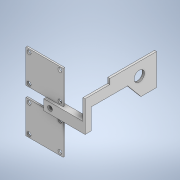
# Autodesk Inventor part: Shelf_half
Saved by Autodesk Inventor 2020.2 (Build 242310000, 310)
## iProperties
Created: 2020-02-18
Part Number: Shelf_half
Material: Generic
Document SubType Name: Modeling
Designer: ColinP
Density: 1 g/cm^3
Appearance: Default
Author: ColinP
Autodesk Inventor part; units mm, degrees
ref_plane "YZ Plane" through (0, 0, 0) normal (1, 0, 0) x (0, 1, 0)
ref_plane "XZ Plane" through (0, 0, 0) normal (0, 1, 0) x (-1, 0, 0)
ref_plane "XY Plane" through (0, 0, 0) normal (0, 0, 1) x (1, 0, 0)
sketch "Sketch14" plane through (0, 0, 0) normal (0, 0, 1) x (1, 0, 0)
  line L0 (0, 0) -> (-6.08, 0)
  line L1 (-6.08, 0) -> (0, 0)
  line L2 (0, 0) -> (6.08, 0)
  line L3 (-6.08, 0) -> (-6.08, 5)
  line L4 (-6.08, 0) -> (-1.08, 0) construction
  line L5 (-6.08, 5) -> (6.08, 5)
  line L6 (6.08, 5) -> (6.08, -5)
  line L7 (6.08, -5) -> (-6.08, -5)
  line L8 (-6.08, -5) -> (-6.08, 5)
  dimension "d66" = 6.08
  dimension "d67" = 6.08
  dimension "d68" = 5
  dimension "d69" = 90
  dimension "d70" = 12.16
  dimension "d71" = 10
  constraints: 18 end point, 3 equal length, 3 horizontal, 2 perpendicular, 1 point on line, 1 vertical
  measures "d66" distance of L0.start L0.end
  measures "d67" distance of L0.start L2.end
  measures "d68" distance of L0.end L3.end
  measures "d69" angle of L4 L3
  measures "d70" distance of L6.end L7.end
  measures "d71" distance of L5.end L6.end
extrude "Extrusion7" add sketch "Sketch14" along normal blind 2
sketch "Sketch15" plane through (0, 0, 2) normal (0, 0, 1) x (1, 0, 0)
  circle A0 centre (0, 0) radius 1.0665
  constraints: 1 centre point, 1 coincident
hole "Hole4" at (0, 0, 2) direction (0, 0, -1) diameter 4.5 end through all clearance for "Flat Head Machine Screw" size "M4" standard "Ansi Metric M Profile"
sketch "Sketch16" plane through (0, 0, 2) normal (0, 0, 1) x (1, 0, 0)
  line L0 (6.08, 5) -> (-6.08, 5) projected
  line L1 (0, 5) -> (10, 5)
  line L2 (10, 5) -> (-25.7, 5)
  line L3 (-25.7, 5) -> (-25.7, 37.05)
  line L4 (-25.7, 37.05) -> (10, 37.05)
  line L5 (10, 37.05) -> (10, 5)
  line L6 (-6.08, -5) -> (6.08, -5) projected
  line L7 (0, -5) -> (10, -5)
  line L8 (10, -5) -> (-25.7, -5)
  line L9 (-25.7, -5) -> (-25.7, -37.05)
  line L10 (-25.7, -37.05) -> (10, -37.05)
  line L11 (10, -37.05) -> (10, -5)
  line L12 (-25.7, 37.05) -> (-22.7, 37.05)
  line L13 (-22.7, 37.05) -> (-22.7, 34.05)
  line L14 (-22.7, 34.05) -> (-25.7, 34.05)
  line L15 (-25.7, 34.05) -> (-25.7, 37.05)
  line L16 (-22.7, 34.05) -> (7, 34.05)
  line L17 (7, 34.05) -> (7, 8)
  line L18 (7, 8) -> (-22.7, 8)
  line L19 (-22.7, 8) -> (-22.7, 34.05)
  line L20 (-25.7, -37.05) -> (-22.7, -37.05)
  line L21 (-22.7, -37.05) -> (-22.7, -34.05)
  line L22 (-22.7, -34.05) -> (-25.7, -34.05)
  line L23 (-25.7, -34.05) -> (-25.7, -37.05)
  line L24 (-22.7, -34.05) -> (7, -34.05)
  line L25 (7, -34.05) -> (7, -8)
  line L26 (7, -8) -> (-22.7, -8)
  line L27 (-22.7, -8) -> (-22.7, -34.05)
  line L28 (-25.7, -5) -> (10, -5)
  line L29 (10, -5) -> (10, -37.05)
  line L30 (10, -37.05) -> (-25.7, -37.05)
  line L31 (-25.7, -37.05) -> (-25.7, -5)
  point P0 (0, 0)
  dimension "d81" = 10
  dimension "d82" = 35.7
  dimension "d83" = 32.05
  dimension "d84" = 35.7
  dimension "d85" = 32.05
  dimension "d86" = 3
  dimension "d87" = 3
  dimension "d88" = 29.7
  dimension "d89" = 26.05
  dimension "d90" = 3
  dimension "d91" = 3
  dimension "d92" = 29.7
  dimension "d93" = 26.05
  dimension "d172" = 10
  constraints: 60 end point, 14 parallel, 9 horizontal, 7 perpendicular, 2 midpoint
  measures "d81" distance of L1.start L1.end
  measures "d82" distance of L3.end L4.end
  measures "d83" distance of L2.end L3.end
  measures "d84" distance of L10.end L9.end
  measures "d85" distance of L9.end L8.end
  measures "d86" distance of L13.end L14.end
  measures "d87" distance of L12.end L13.end
  measures "d88" distance of L17.end L18.end
  measures "d89" distance of L16.end L17.end
  measures "d90" distance of L22.end L21.end
  measures "d91" distance of L21.end L20.end
  measures "d92" distance of L26.end L25.end
  measures "d93" distance of L25.end L24.end
  measures "d172" distance from line of L7.start L11
extrude "Extrusion8" add sketch "Sketch16" along normal blind 1.5 contours L16 L17 L18 L19 | L0 L2 L3 L14 L13 L4 L5 L1 | L13 L14 L3 L4 | L27 L26 L25 L24 | L6 L7 L11 L10 L21 L22 L9 L8 | L22 L21 L10 L9
hole "Hole5" at (-22.7, 34.05, 2) at (-22.7, 8, 2) at (7, 8, 2) at (7, 34.05, 2) at (7, -8, 2) at (7, -34.05, 2) at (-22.7, -34.05, 2) at (-22.7, -8, 2) direction (0, 0, 1) diameter 3.9 end through all clearance for "Flat Head Machine Screw" size "M3.5" standard "Ansi Metric M Profile"
sketch "Sketch17" plane through (0, 0, 2) normal (0, 0, 1) x (1, 0, 0)
  circle A0 centre (0, 0) radius 2.25 projected
  line L0 (6.08, -5) -> (6.08, 5) projected
  line L1 (6.08, 5) -> (-6.08, 5) projected
  line L2 (-6.08, 5) -> (-6.08, -5) projected
  line L3 (-6.08, -5) -> (6.08, -5) projected
extrude "Extrusion9" add sketch "Sketch17" along normal blind 4
sketch "Sketch18" plane through (6.08, -5, 0) normal (1, 0, 0) x (0, 0, -1)
  line L0 (0, 0) -> (0, 10) projected
  line L1 (0, 10) -> (-2, 10) projected
  line L2 (-3.5, 10) -> (-2, 10) projected
  line L3 (-3.5, 10) -> (-6, 10) projected
  line L4 (-6, 0) -> (-6, 10) projected
  line L5 (-3.5, 0) -> (-6, 0) projected
  line L6 (-2, 0) -> (-3.5, 0) projected
  line L7 (0, 0) -> (-2, 0) projected
  point P0 (0, 5)
extrude "Extrusion10" add sketch "Sketch18" along normal blind 35
sketch "Sketch19" plane through (41.08, -5, 0) normal (1, 0, 0) x (0, 0, -1)
  line L0 (-6, 10) -> (-6, 0) projected
  line L1 (-6, 0) -> (-16, 0)
  line L2 (-16, 0) -> (-16, 50)
  line L3 (-16, 50) -> (29, 50)
  line L4 (29, 50) -> (29, 25)
  line L5 (29, 25) -> (0, 10)
  line L6 (0, 10) -> (0, 0) projected
  line L7 (0, 10) -> (0, 0)
  line L8 (0, 0) -> (-6, 0)
  point P0 (0, 5)
  dimension "d107" = 10
  dimension "d108" = 50
  dimension "d109" = 90
  dimension "d110" = 45
  dimension "d111" = 90
  dimension "d112" = 25
  constraints: 14 end point, 3 perpendicular, 1 horizontal, 1 parallel, 1 vertical
  measures "d107" distance of L0.end L1.end
  measures "d108" distance of L1.end L2.end
  measures "d109" angle of L1 L2
  measures "d110" distance of L2.end L3.end
  measures "d111" angle of L2 L3
  measures "d112" distance of L3.end L4.end
extrude "Extrusion11" add sketch "Sketch19" along normal blind 2.5
sketch "Sketch21" plane through (43.58, -5, 0) normal (1, 0, 0) x (0, 0, -1)
  line L0 (-3.5, 10) -> (-6, 10) projected
  line L1 (0, 10) -> (0, 24.05)
  line L2 (0, 10) -> (14.05, 10) construction
  line L3 (0, 24.05) -> (6.713, 24.05)
  point P0 (0, 5)
  point P1 (3, 10)
  point P2 (-2, 10)
  dimension "d118" = 14.05
  dimension "d119" = 90
  dimension "d120" = 6.713
  dimension "d121" = 90
  constraints: 6 end point, 2 perpendicular, 1 horizontal, 1 point on line, 1 vertical
  measures "d118" distance of L1.start L1.end
  measures "d119" angle of L2 L1
  measures "d120" distance of L1.end L3.end
  measures "d121" angle of L1 L3
hole "Hole6" at (43.58, 19.05, -6.713) direction (-1, 0, 0) diameter 10 end through all
sketch "Sketch22" plane through (43.58, -5, 0) normal (1, 0, 0) x (0, 0, -1)
  circle A0 centre (6.713, 24.05) radius 5 projected
  line L0 (6.713, 24.05) -> (6.713, 32.05)
  line L1 (6.713, 24.05) -> (14.713, 24.05) construction
  line L2 (6.713, 32.05) -> (24.213, 32.05)
  line L3 (24.213, 32.05) -> (-10.787, 32.05)
  point P0 (0, 5)
  dimension "d129" = 8
  dimension "d130" = 90
  dimension "d131" = 17.5
  dimension "d132" = 90
  dimension "d133" = 35
  constraints: 8 end point, 2 perpendicular, 1 horizontal, 1 point on line, 1 vertical
  measures "d129" distance of L0.start L0.end
  measures "d130" angle of L1 L0
  measures "d131" distance of L0.end L2.end
  measures "d132" angle of L0 L2
  measures "d133" distance of L2.end L3.end
hole "Hole7" at (43.58, 27.05, 10.787) at (43.58, 27.05, -24.213) direction (-1, 0, 0) diameter 4.2 end through all
sketch "Sketch23" plane through (43.58, -5, 0) normal (1, 0, 0) x (0, 0, -1)
  line L0 (-3.5, 0) -> (-2, 0) projected
  line L1 (-2, 0) -> (-2, -9)
  line L2 (-2, 0) -> (7, 0) construction
  line L3 (-2, -9) -> (33, -9) construction
  line L4 (-2, -9) -> (33, -9)
  line L5 (-2, -9) -> (33, -9) construction
  line L6 (33, -9) -> (40.7782, -1.2218)
  line L7 (40.7782, -1.2218) -> (60.7782, -1.2218)
  line L8 (33, -9) -> (68, -9)
  line L9 (33, -9) -> (68, -9) construction
  line L10 (68, -9) -> (68, -1.2218)
  line L11 (68, -1.2218) -> (60.7782, -1.2218)
  line L12 (68, -9) -> (68, -29)
  line L13 (68, -9) -> (88, -9) construction
  line L14 (68, -29) -> (-2, -29)
  line L15 (-2, -29) -> (-2, -9)
  line L16 (33, -9) -> (44.45, -9)
  line L17 (44.45, -9) -> (44.45, -13.669)
  line L18 (44.45, -9) -> (49.119, -9) construction
  line L19 (44.45, -13.669) -> (44.45, -21.669)
  line L20 (44.45, -21.669) -> (61.95, -21.669)
  line L21 (61.95, -21.669) -> (26.95, -21.669)
  circle A0 centre (26.95, -21.669) radius 2.1
  circle A1 centre (61.95, -21.669) radius 2.1
  circle A2 centre (44.45, -13.669) radius 5
  point P0 (0, 5)
  dimension "d141" = 9
  dimension "d142" = 90
  dimension "d145" = 35
  dimension "d146" = 0
  dimension "d147" = 11
  dimension "d148" = 135
  dimension "d149" = 20
  dimension "d150" = 35
  dimension "d151" = 0
  dimension "d152" = 20
  dimension "d153" = 90
  dimension "d154" = 90
  dimension "d155" = 11.45
  dimension "d156" = 4.669
  dimension "d157" = 90
  dimension "d158" = 8
  dimension "d159" = 17.5
  dimension "d160" = 35
  dimension "d161" = 4.2
  dimension "d162" = 4.2
  dimension "d163" = 10
  constraints: 42 end point, 8 horizontal, 5 equal length, 4 perpendicular, 3 centre point, 3 coincident, 3 point on line, 3 vertical, 1 parallel
  measures "d141" distance of L0.end L1.end
  measures "d142" angle of L1 L2
  measures "d145" distance of L1.end L3.end
  measures "d146" distance between parallel lines of L4 L5
  measures "d147" distance of L3.end L6.end
  measures "d148" angle of L6 L4
  measures "d149" distance of L6.end L7.end
  measures "d150" distance of L5.end L8.end
  measures "d151" distance between parallel lines of L8 L9
  measures "d152" distance of L8.end L12.end
  measures "d153" angle of L12 L13
  measures "d154" angle of L12 L14
  measures "d155" distance of L5.end L16.end
  measures "d156" distance of L16.end L17.end
  measures "d157" angle of L17 L18
  measures "d158" distance of L17.end L19.end
  measures "d159" distance of L19.end L20.end
  measures "d160" distance of L20.end L21.end
  measures "d161" diameter of A0
  measures "d162" diameter of A1
  measures "d163" diameter of A2
extrude "Extrusion13" add sketch "Sketch23" against normal blind 2 contours L4 L8 A2 L12 L14 L15 | L6 L7 L11 L10 L8 A2
sketch "Sketch24" plane through (43.58, -5, 0) normal (1, 0, 0) x (0, 0, -1)
  line L0 (-16, 50) -> (-16, 0) projected
  line L1 (-16, 0) -> (-16, -29)
  line L2 (68, -29) -> (-2, -29) projected
  line L3 (-16, -29) -> (-2, -29)
  line L4 (0, 0) -> (-2, 0) projected
  line L5 (-2, -29) -> (-2, 0)
  line L6 (-16, 0) -> (0, 0) projected
  line L7 (-2, 0) -> (-16, 0)
  point P0 (0, 5)
  point P1 (3, 0)
  constraints: 8 end point, 3 perpendicular, 1 collinear
extrude "Extrusion14" add sketch "Sketch24" against normal blind 2
sketch "Sketch25" plane through (41.58, -5, 0) normal (-1, 0, 0) x (0, 0, 1)
  line L0 (2, -9) -> (-33, -9) projected
  line L1 (-33, -9) -> (2, -9)
  line L2 (2, -9) -> (2, -11)
  line L3 (2, -11) -> (-33, -11)
  line L4 (-33, -11) -> (-33, -9)
  line L5 (2, -11) -> (6, -11)
  line L6 (6, -11) -> (6, 0)
  line L7 (6, 0) -> (2, 0)
  line L8 (2, 0) -> (2, -11)
  point P0 (0, 5)
  point P1 (2, -9)
  dimension "d168" = 35
  dimension "d169" = 2
  constraints: 16 end point, 4 parallel, 2 horizontal, 2 perpendicular
  measures "d168" distance of L2.end L3.end
  measures "d169" distance of L1.end L2.end
extrude "Extrusion15" add sketch "Sketch25" along normal blind 10
sketch "Sketch27" plane through (43.58, -5, 0) normal (1, 0, 0) x (0, 0, -1)
  line L0 (68, -29) -> (-16, -29) projected
  line L1 (-16, -29) -> (69.4034, -29)
  line L2 (69.4034, -29) -> (69.4034, 52.4533)
  line L3 (69.4034, 52.4533) -> (-16, 52.4533)
  line L4 (-16, 52.4533) -> (-16, -29)
  point P0 (0, 5)
  constraints: 8 end point, 2 parallel, 1 horizontal, 1 perpendicular
extrude "Extrusion17" cut sketch "Sketch27" against normal up to surface (12 mm away)
sketch "Sketch28" plane through (0, 0, 0) normal (0, 0, -1) x (-1, 0, 0)
  line L0 (6.08, -5) -> (-10, -5) projected
  line L1 (6.08, 5) -> (-10, 5) projected
  line L2 (6.08, -5) -> (5.08, -5)
  line L3 (5.08, -5) -> (5.08, 5)
  line L4 (5.08, 5) -> (6.08, 5)
  line L5 (6.08, 5) -> (6.08, -5)
  point P0 (0, 0)
  dimension "d177" = 1
  constraints: 8 end point, 2 parallel, 1 horizontal, 1 perpendicular, 1 point on line
  measures "d177" distance of L3.end L4.end
extrude "Extrusion18" add sketch "Sketch28" along normal blind 5
sketch "Sketch29" plane through (31.58, -5, 6) normal (1, 0, 0) x (0, 0, -1)
  line L0 (6, 10) -> (6, 20)
  line L1 (6, 20) -> (41, 20)
  line L2 (6, 20) -> (41, 20) construction
  line L3 (41, 20) -> (53.8558, 4.6791)
  line L4 (53.8558, 4.6791) -> (68.8558, 4.6791)
  line L5 (68.8558, 4.6791) -> (68.8558, 34.6791)
  line L6 (68.8558, 34.6791) -> (23.8558, 34.6791)
  line L7 (68.8558, 34.6791) -> (113.8558, 34.6791) construction
  line L8 (23.8558, 34.6791) -> (23.8558, 29.6791)
  line L9 (0, 10) -> (0, 0) projected
  line L10 (0, 10) -> (0, 29.6791)
  line L11 (0, 29.6791) -> (23.8558, 29.6791)
  line L12 (6, 10) -> (6, 0)
  line L13 (6, 0) -> (0, 0)
  line L14 (0, 0) -> (0, 10)
  point P0 (6, 5)
  dimension "d180" = 10
  dimension "d181" = 35
  dimension "d182" = 0
  dimension "d183" = 20
  dimension "d184" = 130
  dimension "d185" = 15
  dimension "d186" = 30
  dimension "d187" = 45
  dimension "d188" = 180
  dimension "d189" = 5
  dimension "d190" = 90
  constraints: 28 end point, 5 perpendicular, 4 horizontal, 3 vertical, 2 collinear, 1 parallel
  measures "d180" distance of L0.start L0.end
  measures "d181" distance of L0.end L1.end
  measures "d182" distance between parallel lines of L1 L2
  measures "d183" distance of L1.end L3.end
  measures "d184" angle of L1 L3
  measures "d185" distance of L3.end L4.end
  measures "d186" distance of L4.end L5.end
  measures "d187" distance of L5.end L6.end
  measures "d188" angle of L6 L7
  measures "d189" distance of L6.end L8.end
  measures "d190" angle of L8 L6
extrude "Extrusion19" add sketch "Sketch29" along normal blind 2
sketch "Sketch30" plane through (33.58, -5, 6) normal (1, 0, 0) x (0, 0, -1)
  line L0 (68.8558, 4.6791) -> (68.8558, 34.6791) projected
  line L1 (68.8558, 34.6791) -> (52.1638, 34.6791)
  line L2 (68.8558, 34.6791) -> (23.8558, 34.6791) projected
  line L3 (52.1638, 34.6791) -> (52.1638, 22.4901)
  circle A0 centre (52.1638, 22.4901) radius 5
  point P0 (6, 5)
  dimension "d193" = 16.692
  dimension "d194" = 12.189
  dimension "d195" = 10
  constraints: 4 end point, 1 centre point, 1 coincident, 1 point on line, 1 vertical
  measures "d193" distance of L0.end L1.end
  measures "d194" distance of L1.end L3.end
  measures "d195" diameter of A0
extrude "Extrusion20" cut sketch "Sketch30" against normal blind 10
body "Solid2"
